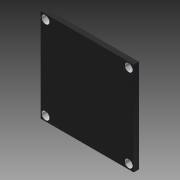
# Autodesk Inventor part: FC 36x36
Saved by Autodesk Inventor 2015 (Build 190159000, 159)
## iProperties
Created: 2016-11-27
Part Number: FC 36x36
Material: Generic
Document SubType Name: Modeling
Designer: Hampus
Density: 1 g/cm^3
Appearance: Rubber - Black
Author: Hampus
Autodesk Inventor part; units mm, degrees
ref_plane "YZ Plane" through (0, 0, 0) normal (1, 0, 0) x (0, 1, 0)
ref_plane "XZ Plane" through (0, 0, 0) normal (0, 1, 0) x (-1, 0, 0)
ref_plane "XY Plane" through (0, 0, 0) normal (0, 0, 1) x (1, 0, 0)
sketch "Sketch1" plane through (0, 0, 0) normal (0, 1, 0) x (-1, 0, 0)
  line L0 (0, 0) -> (-36, 0)
  line L1 (-36, 0) -> (-36, -36)
  line L2 (-36, -36) -> (0, -36)
  line L3 (0, -36) -> (0, 0)
  circle A0 centre (-1.9445, -34.0555) radius 1.5
  circle A1 centre (-34.0555, -34.0555) radius 1.5
  circle A2 centre (-1.9445, -1.9445) radius 1.5
  circle A3 centre (-34.0555, -1.9445) radius 1.5
  line L4 (-10.5351, -31.1412) -> (-23.3582, -31.1412)
  line L5 (-23.3582, -31.1412) -> (-23.3582, -27.4511)
  line L6 (-23.3582, -27.4511) -> (-10.5351, -27.4511)
  line L7 (-10.5351, -27.4511) -> (-10.5351, -31.1412)
  line L8 (-9.059, -24.6835) -> (-4.3542, -24.6835)
  line L9 (-4.3542, -24.6835) -> (-4.3542, -15.1815)
  line L10 (-4.3542, -15.1815) -> (-9.059, -15.1815)
  line L11 (-9.059, -15.1815) -> (-9.059, -24.6835)
  line L12 (-9.059, -9.1851) -> (-14.6864, -9.1851)
  line L13 (-14.6864, -9.1851) -> (-14.6864, -4.2957)
  line L14 (-14.6864, -4.2957) -> (-9.059, -4.2957)
  line L15 (-9.059, -4.2957) -> (-9.059, -9.1851)
  line L16 (-12.3801, -22.1005) -> (-25.2032, -22.1005)
  line L17 (-25.2032, -22.1005) -> (-25.2032, -13.3365)
  line L18 (-25.2032, -13.3365) -> (-12.3801, -13.3365)
  line L19 (-12.3801, -13.3365) -> (-12.3801, -22.1005)
  line L20 (-23.3582, -8.5394) -> (-29.1701, -8.5394)
  line L21 (-29.1701, -8.5394) -> (-29.1701, -3.4445)
  line L22 (-29.1701, -3.4445) -> (-23.3582, -3.4445)
  line L23 (-23.3582, -3.4445) -> (-23.3582, -8.5394)
  line L24 (-32.5555, -15.1815) -> (-29.1701, -15.1815)
  line L25 (-29.1701, -15.1815) -> (-29.1701, -21.2702)
  line L26 (-29.1701, -21.2702) -> (-32.5555, -21.2702)
  line L27 (-32.5555, -21.2702) -> (-32.5555, -15.1815)
  line L28 (-30.8628, -27.4511) -> (-29.1701, -27.4511)
  line L29 (-29.1701, -27.4511) -> (-29.1701, -25.9751)
  line L30 (-29.1701, -25.9751) -> (-30.8628, -25.9751)
  line L31 (-30.8628, -25.9751) -> (-30.8628, -27.4511)
  line L32 (-25.2032, -25.9751) -> (-23.3582, -25.9751)
  line L33 (-23.3582, -25.9751) -> (-23.3582, -24.6835)
  line L34 (-23.3582, -24.6835) -> (-25.2032, -24.6835)
  line L35 (-25.2032, -24.6835) -> (-25.2032, -25.9751)
  line L36 (-16.9466, -25.9751) -> (-15.609, -25.9751)
  line L37 (-15.609, -25.9751) -> (-15.609, -23.8533)
  line L38 (-15.609, -23.8533) -> (-16.9466, -23.8533)
  line L39 (-16.9466, -23.8533) -> (-16.9466, -25.9751)
  line L40 (-6.7066, -31.1412) -> (-5.2767, -31.1412)
  line L41 (-5.2767, -31.1412) -> (-5.2767, -29.2962)
  line L42 (-5.2767, -29.2962) -> (-6.7066, -29.2962)
  line L43 (-6.7066, -29.2962) -> (-6.7066, -31.1412)
  line L44 (-7.214, -11.6759) -> (-1.9445, -11.6759)
  line L45 (-1.9445, -11.6759) -> (-1.9445, -10.5689)
  line L46 (-1.9445, -10.5689) -> (-7.214, -10.5689)
  line L47 (-7.214, -10.5689) -> (-7.214, -11.6759)
  dimension "d0" = 36
  dimension "d1" = 36
  dimension "d4" = 3
  dimension "d5" = 3
  constraints: 96 end point, 24 parallel, 12 horizontal, 12 perpendicular, 12 point on line, 4 centre point
  measures "d0" distance of L2.end L1.end
  measures "d1" distance of L1.end L0.end
  measures "d4" diameter of A0
  measures "d5" diameter of A1
extrude "Extrusion1" add sketch "Sketch1" along normal blind 2 contours L3 L2 L1 L0 | L4 L5 L6 L7 | L11 L10 L9 L8 | L12 L13 L14 L15 | L16 L17 L18 L19 | L20 L21 L22 L23 | L24 L25 L26 L27 | L31 L30 L29 L28 | L35 L34 L33 L32 | L39 L38 L37 L36 | L43 L42 L41 L40 | L47 L46 L45 L44
extrude "Extrusion2" add sketch "Sketch1" along normal blind 2.2 contours L4 L5 L6 L7 | L11 L10 L9 L8 | L12 L13 L14 L15 | L16 L17 L18 L19 | L20 L21 L22 L23 | L24 L25 L26 L27 | L31 L30 L29 L28 | L35 L34 L33 L32 | L39 L38 L37 L36 | L43 L42 L41 L40 | L47 L46 L45 L44
body "Solid1"
